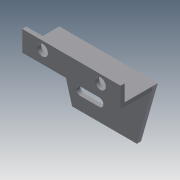
# Autodesk Inventor part: ruka_paka
Saved by Autodesk Inventor 2013 (Build 170138000, 138)
## iProperties
Created: 2013-03-08
Part Number: ruka_paka
Material: Generic
Document SubType Name: Modeling
Designer: idle-rug
Density: 1 g/cm^3
Author: idle-rug
Autodesk Inventor part; units mm, degrees
ref_plane "YZ Plane" through (0, 0, 0) normal (1, 0, 0) x (0, 1, 0)
ref_plane "XZ Plane" through (0, 0, 0) normal (0, 1, 0) x (-1, 0, 0)
ref_plane "XY Plane" through (0, 0, 0) normal (0, 0, 1) x (1, 0, 0)
sketch "Sketch1" plane through (0, 0, 0) normal (0, 0, 1) x (1, 0, 0)
  line L0 (18, 6.05) -> (-18, 6.05)
  line L1 (-18, 6.05) -> (-18, -6.05)
  line L2 (-18, -6.05) -> (18, -6.05)
  line L3 (18, -6.05) -> (18, 6.05)
  line L4 (18, 6.05) -> (-18, -6.05) construction
  line L5 (-18, 6.05) -> (18, -6.05) construction
  point P0 (0, 0)
  dimension "d0" = 36
  dimension "d1" = 12.1
  constraints: 12 end point, 2 midpoint, 2 parallel, 1 horizontal, 1 perpendicular
  measures "d0" distance of L2.end L1.end
  measures "d1" distance of L1.end L0.end
extrude "Extrusion1" add sketch "Sketch1" along normal blind 1.5
sketch "Sketch2" plane through (0, 0, 0) normal (0, 0, -1) x (-1, 0, 0)
  line L0 (-18, 6.05) -> (18, 6.05) projected
  line L1 (-18, -6.05) -> (-18, 6.05) projected
  line L2 (18, 6.05) -> (18, -6.05) projected
  line L3 (-18, 6.05) -> (-18, 4.55)
  line L4 (-18, 4.55) -> (18, 4.55)
  line L5 (18, 4.55) -> (18, 6.05)
  line L6 (18, 6.05) -> (-18, 6.05)
  point P0 (0, 0)
  dimension "d4" = 1.5
  constraints: 8 end point, 2 collinear, 2 point on line, 1 perpendicular
  measures "d4" distance of L0.start L3.end
extrude "Extrusion2" add sketch "Sketch2" along normal blind 30
sketch "Sketch3" plane through (-18, -6.05, 0) normal (0, -1, 0) x (1, 0, 0)
  line L0 (0, 0) -> (36, 0) projected
  line L1 (36, 0) -> (36, 1.5) projected
  line L2 (0, 1.5) -> (36, 1.5) projected
  line L3 (0, 0) -> (0, 1.5) projected
  point P0 (18, 0)
extrude "Extrusion3" add sketch "Sketch3" along normal blind 1.5
sketch "Sketch4" plane through (0, 0, 1.5) normal (0, 0, 1) x (1, 0, 0)
  line L0 (-18, 6.05) -> (-18, -7.55) projected
  line L1 (18, -7.55) -> (-18, -7.55) projected
  line L2 (18, 6.05) -> (18, -7.55) projected
  line L3 (-18, -7.55) -> (-18, -6.05)
  line L4 (-18, -6.05) -> (18, -6.05)
  line L5 (18, -7.55) -> (18, -6.05)
  line L6 (18, -7.55) -> (-18, -7.55)
  point P0 (0, 0)
  dimension "d9" = 1.5
  constraints: 8 end point, 2 collinear, 2 point on line, 1 perpendicular
  measures "d9" distance of L0.end L3.end
extrude "Extrusion4" add sketch "Sketch4" along normal blind 6
sketch "Sketch5" plane through (-18, 6.05, 1.5) normal (0, 1, 0) x (1, 0, 0)
  line L0 (0, 31.5) -> (36, 31.5) projected
  line L1 (18, 31.5) -> (18, 26.5)
  line L2 (18, 26.5) -> (14.5, 26.5)
  line L3 (18, 26.5) -> (21.5, 26.5)
  circle A0 centre (14.5, 26.5) radius 1.5
  circle A1 centre (21.5, 26.5) radius 1.5
  line L4 (14.5, 25) -> (21.5, 25)
  line L5 (14.5, 28) -> (21.5, 28)
  point P0 (18, 1.5)
  dimension "d12" = 5
  dimension "d13" = 3.5
  dimension "d14" = 3.5
  dimension "d15" = 3
  dimension "d16" = 3
  constraints: 10 end point, 4 point on circle, 2 centre point, 2 coincident, 2 perpendicular, 2 tangent, 1 collinear, 1 midpoint
  measures "d12" distance of L1.start L1.end
  measures "d13" distance of L1.end L2.end
  measures "d14" distance of L1.end L3.end
  measures "d15" diameter of A0
  measures "d16" diameter of A1
extrude "Extrusion5" cut sketch "Sketch5" against normal blind 2
sketch "Sketch6" plane through (-18, 6.05, 1.5) normal (0, 1, 0) x (1, 0, 0)
  line L0 (0, 31.5) -> (0, 0) projected
  line L1 (36, 0) -> (36, 31.5) projected
  line L2 (0, 31.5) -> (36, 31.5) projected
  line L3 (0, 31.5) -> (9, 31.5)
  line L4 (9, 31.5) -> (0, 0)
  line L5 (0, 0) -> (0, 31.5)
  line L6 (36, 31.5) -> (27, 31.5)
  line L7 (27, 31.5) -> (36, 0)
  line L8 (36, 0) -> (36, 31.5)
  point P0 (18, 1.5)
  dimension "d19" = 9
  dimension "d20" = 9
  constraints: 12 end point, 2 collinear, 2 point on line
  measures "d19" distance of L0.start L3.end
  measures "d20" distance of L1.end L6.end
extrude "Extrusion6" cut sketch "Sketch6" against normal blind 2
sketch "Sketch7" plane through (-18, -6.05, 1.5) normal (0, 1, 0) x (1, 0, 0)
  line L0 (36, -6) -> (0, -6) projected
  line L1 (36, 0) -> (36, -6) projected
  line L2 (18, -6) -> (18, -3)
  circle A0 centre (18, -3) radius 2
  circle A1 centre (4.907, -3) radius 1.5
  circle A2 centre (31.093, -3) radius 1.5
  point P0 (18, 1.5)
  dimension "d23" = 4
  dimension "d25" = 3
  dimension "d26" = 3
  constraints: 3 centre point, 2 end point, 1 coincident, 1 midpoint, 1 parallel
  measures "d23" diameter of A0
  measures "d25" diameter of A1
  measures "d26" diameter of A2
extrude "Extrusion7" cut sketch "Sketch7" against normal blind 2
sketch "Sketch8" plane through (-18, -6.05, 1.5) normal (0, 1, 0) x (1, 0, 0)
  circle A0 centre (18, -3) radius 2 projected
  circle A1 centre (18, -3) radius 10.593
  circle A2 centre (7.407, -3) radius 2
  circle A3 centre (28.593, -3) radius 2
  point P0 (18, 1.5)
  dimension "d29" = 21.186
  dimension "d30" = 4
  dimension "d31" = 4
  constraints: 3 centre point, 2 point on circle, 1 coincident
  measures "d29" diameter of A1
  measures "d30" diameter of A2
  measures "d31" diameter of A3
extrude "Extrusion8" cut sketch "Sketch8" against normal blind 1.5 contours A1 A3 | A1 A3 | A2 A1 | A1 A2
sketch "Sketch9" plane through (-18, -6.05, 1.5) normal (0, 1, 0) x (1, 0, 0)
  circle A0 centre (18, -3) radius 2 projected
  arc A1 (5.807, -4.2) -> (5.807, -1.8) centre (7.407, -3) ccw projected
  arc A2 (5.807, -1.8) -> (5.807, -4.2) centre (4.907, -3) ccw projected
  arc A3 (30.193, -1.8) -> (30.193, -4.2) centre (28.593, -3) ccw projected
  arc A4 (30.193, -4.2) -> (30.193, -1.8) centre (31.093, -3) ccw projected
  circle A5 centre (7.407, -3) radius 2
  circle A6 centre (28.593, -3) radius 2
  point P0 (18, 1.5)
  constraints: 2 coincident, 6 other
extrude "Extrusion9" add sketch "Sketch9" against normal blind 1.5 contours A0 | A2 A5 | A4 A6
sketch "Sketch10" plane through (-18, 6.05, 1.5) normal (0, 1, 0) x (1, 0, 0)
  line L0 (9, 31.5) -> (0, 0) projected
  line L1 (36, 0) -> (0, 0) projected
  line L2 (36, 0) -> (27, 31.5) projected
  line L3 (9, 31.5) -> (27, 31.5) projected
  line L4 (18, 31.5) -> (18, 21.5)
  line L5 (18, 21.5) -> (6.1429, 21.5)
  line L6 (18, 21.5) -> (29.8571, 21.5)
  line L7 (6.1429, 21.5) -> (9, 31.5)
  line L8 (9, 31.5) -> (27, 31.5)
  line L9 (27, 31.5) -> (29.8571, 21.5)
  point P0 (18, 1.5)
  dimension "d36" = 10
  constraints: 12 end point, 4 collinear, 2 perpendicular, 2 point on line, 1 midpoint
  measures "d36" distance of L4.start L4.end
extrude "Extrusion10" cut sketch "Sketch10" against normal blind 1.5 contours L3 L4 L5 L0 | L3 L2 L6 L4
sketch "Sketch11" plane through (-18, 6.05, 1.5) normal (0, 1, 0) x (1, 0, 0)
  line L0 (29.8571, 21.5) -> (6.1429, 21.5) projected
  line L1 (18, 21.5) -> (12.6, 21.5)
  line L2 (12.6, 21.5) -> (12.6, 15.2)
  line L3 (12.6, 15.2) -> (9.1, 15.2)
  line L4 (9.1, 15.2) -> (16.1, 15.2)
  circle A0 centre (9.1, 15.2) radius 1.5
  circle A1 centre (16.1, 15.2) radius 1.5
  line L5 (9.1, 16.7) -> (16.1, 16.7)
  line L6 (16.1, 13.7) -> (9.1, 13.7)
  point P0 (18, 1.5)
  dimension "d39" = 5.4
  dimension "d40" = 6.3
  dimension "d41" = 3.5
  dimension "d42" = 7
  dimension "d43" = 3
  dimension "d44" = 3
  constraints: 12 end point, 4 point on circle, 3 tangent, 2 centre point, 2 coincident, 2 perpendicular, 1 collinear, 1 midpoint, 1 point on line
  measures "d39" distance of L1.start L1.end
  measures "d40" distance of L1.end L2.end
  measures "d41" distance of L2.end L3.end
  measures "d42" distance of L3.end L4.end
  measures "d43" diameter of A0
  measures "d44" diameter of A1
extrude "Extrusion11" cut sketch "Sketch11" against normal blind 1.5
body "Solid1"
